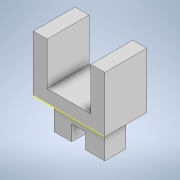
# Autodesk Inventor part: servo_motor_clip
Saved by Autodesk Inventor 2022 (Build 260153000, 153)
## iProperties
Created: 2024-03-21
Part Number: servo_motor_clip
Material: Generic
Document SubType Name: Modeling
Designer: subin
Density: 1 g/cm^3
Appearance: Default
Author: subin
Autodesk Inventor part; units mm, degrees
ref_plane "YZ Plane" through (0, 0, 0) normal (1, 0, 0) x (0, 1, 0)
ref_plane "XZ Plane" through (0, 0, 0) normal (0, 1, 0) x (-1, 0, 0)
ref_plane "XY Plane" through (0, 0, 0) normal (0, 0, 1) x (1, 0, 0)
sketch "Sketch1" plane through (0, 0, 0) normal (0, 0, 1) x (1, 0, 0)
  line L0 (-0.1073, 3.7083) -> (12.3927, 3.7083)
  line L1 (12.3927, 3.7083) -> (12.3927, 0)
  line L2 (12.3927, 0) -> (-0.1073, 0)
  line L3 (-0.1073, 0) -> (-0.1073, 3.7083)
  line L4 (-0.1073, 0) -> (-4.1073, 0)
  line L5 (-4.1073, 0) -> (-4.1073, 16)
  line L6 (-4.1073, 16) -> (-0.1073, 16)
  line L7 (-0.1073, 16) -> (-0.1073, 0)
  line L8 (12.3927, 0) -> (16.3927, 0)
  line L9 (16.3927, 0) -> (16.3927, 16)
  line L10 (16.3927, 16) -> (12.3927, 16)
  line L11 (12.3927, 16) -> (12.3927, 0)
  point P0 (0, 0)
  dimension "d0" = 12.5
  dimension "d1" = 16
  dimension "d2" = 4
  dimension "d3" = 4
  constraints: 24 end point, 6 parallel, 3 horizontal, 3 perpendicular, 1 point on line
  measures "d0" distance of L1.end L2.end
  measures "d1" distance of L4.end L5.end
  measures "d2" distance of L5.end L6.end
  measures "d3" distance of L9.end L10.end
extrude "Extrusion1" add sketch "Sketch1" along normal blind 12
sketch "Sketch2" plane through (-4.1073, 0, 0) normal (0, -1, 0) x (1, 0, 0)
  line L0 (0, 12) -> (20.5, 12) projected
  line L1 (0, 0) -> (20.5, 0) projected
  line L2 (0, 0) -> (0, 12) projected
  point P0 (4.1073, 0)
sketch "Sketch3" plane through (-4.1073, 0, 0) normal (0, -1, 0) x (1, 0, 0)
  line L0 (17.5, 3) -> (17.5, 9)
  line L1 (0, 0) -> (20.5, 0) projected
  line L2 (0, 0) -> (0, 12) projected
  line L3 (20.5, 0) -> (20.5, 12) projected
  line L4 (17.5, 3) -> (3, 3)
  line L5 (3, 3) -> (3, 9)
  line L6 (3, 9) -> (17.5, 9)
  line L7 (17.5, 9) -> (17.5, 3)
  point P0 (4.1073, 0)
  dimension "d20" = 3
  dimension "d21" = 3
  constraints: 10 end point, 2 parallel, 1 horizontal, 1 perpendicular
  measures "d20" distance between parallel lines of L2 L5
  measures "d21" distance between parallel lines of L3 L0
extrude "Extrusion4" add sketch "Sketch3" along normal blind 4.5
sketch "Sketch5" plane through (-4.1073, -4.5, 0) normal (0, -1, 0) x (1, 0, 0)
  line L0 (3, 3) -> (17.5, 3) projected
  line L1 (3, 9) -> (17.5, 9) projected
  line L2 (17.5, 3) -> (12, 3)
  line L3 (12, 3) -> (12, 9)
  line L4 (12, 9) -> (17.5, 9)
  line L5 (17.5, 9) -> (17.5, 3)
  line L6 (3, 3) -> (8, 3)
  line L7 (8, 3) -> (8, 9)
  line L8 (8, 9) -> (3, 9)
  line L9 (3, 9) -> (3, 3)
  point P0 (4.1073, 0)
  dimension "d24" = 4
  dimension "d25" = 5.5
  constraints: 16 end point, 4 parallel, 3 point on line, 2 horizontal, 2 perpendicular
  measures "d24" distance between parallel lines of L7 L3
  measures "d25" distance between parallel lines of L5 L3
extrude "Extrusion5" add sketch "Sketch5" along normal blind 4.5 contours L9 L1 L7 L0 | L3 L1 L5 L0
body "Solid1"
